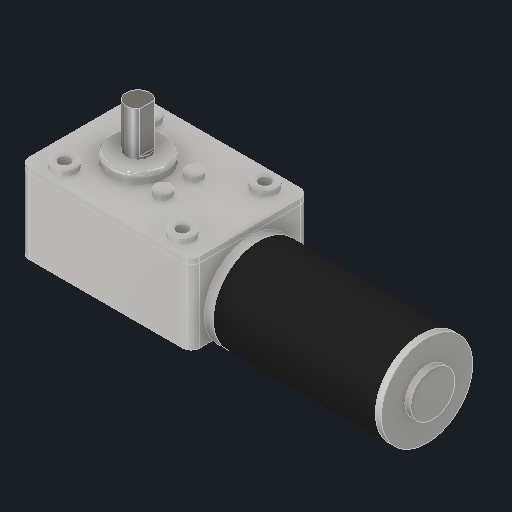
# Autodesk Inventor part: Worm_Gear_Motor_12V
Saved by Autodesk Inventor 2026.2 (Build 302298010, 298A)
## iProperties
Created: 2017-09-17
Part Number: Worm_Gear_Motor_12V
Material: Generic
Document SubType Name: Modeling
Designer: joeyt
Density: 1 g/cm^3
Appearance: Default
Author: joeyt
Autodesk Inventor part; units mm, degrees
ref_plane "YZ Plane" through (0, 0, 0) normal (1, 0, 0) x (0, 1, 0)
ref_plane "XZ Plane" through (0, 0, 0) normal (0, 1, 0) x (-1, 0, 0)
ref_plane "XY Plane" through (0, 0, 0) normal (0, 0, 1) x (1, 0, 0)
sketch "Sketch1" plane through (0, 0, 0) normal (0, 1, 0) x (-1, 0, 0)
  line L0 (-29, 20) -> (29, 20)
  line L1 (29, 20) -> (29, -20)
  line L2 (29, -20) -> (-29, -20)
  line L3 (-29, -20) -> (-29, 20)
  line L4 (-29, 20) -> (29, -20) construction
  line L5 (29, 20) -> (-29, -20) construction
  point P0 (0, 0)
  dimension "d0" = 58
  dimension "d1" = 40
  constraints: 12 end point, 2 midpoint, 2 parallel, 1 horizontal, 1 perpendicular
  measures "d0" distance of L1.end L2.end
  measures "d1" distance of L0.end L1.end
extrude "Extrusion1" add sketch "Sketch1" along normal blind 27
sketch "Sketch2" plane through (0, 27, 0) normal (0, 1, 0) x (1, 0, 0)
  line L0 (-29, 20) -> (-29, -20) projected
  line L1 (0, 0) -> (-29, 0)
  point P0 (-20, 14)
  point P1 (20, 14)
  point P2 (20, -14)
  point P3 (-20, -14)
  dimension "d4" = 40
  dimension "d5" = 28
  dimension "d6" = 9
  constraints: 2 end point, 2 horizontal alignment, 2 vertical alignment, 1 midpoint, 1 symmetric about line
  measures "d4" distance of point (20, 14) point (-20, 14)
  measures "d5" distance of point (-20, -14) point (-20, 14)
  measures "d6" distance from line of L0 point (-20, 14)
sketch "Sketch3" plane through (0, 27, 0) normal (0, 1, 0) x (1, 0, 0)
  circle A0 centre (-20, 14) radius 4
  circle A1 centre (-20, 14) radius 2
  point P0 (0, 0)
  dimension "d7" = 8
  dimension "d8" = 4
  constraints: 2 centre point, 2 coincident
  measures "d7" diameter of A0
  measures "d8" diameter of A1
extrude "Extrusion2" add sketch "Sketch3" along normal blind 2
sketch "Sketch11" plane through (-20, 27, -14) normal (0, 1, 0) x (1, 0, 0)
  circle A0 centre (0, 0) radius 2 projected
  point P0 (20, -14)
extrude "Extrusion9" cut sketch "Sketch11" against normal blind 10
pattern_sketch "Sketch Driven Pattern1" of "Extrusion2", "Extrusion9" from (-20, 27, -14) copies at (20, 27, -14) at (20, 27, 14) at (-20, 27, 14)
sketch "Sketch4" plane through (0, 27, 0) normal (0, 1, 0) x (1, 0, 0)
  circle A0 centre (-20, 14) radius 2 projected
  circle A1 centre (-20, -14) radius 2 projected
  circle A2 centre (-20, 14) radius 4 projected
  line L0 (-20, 14) -> (-20, -14)
  line L1 (-20, 0) -> (-9, 0)
  circle A3 centre (-9, 0) radius 9.5
  point P0 (0, 0)
  dimension "d11" = 11
  dimension "d12" = 19
  constraints: 4 end point, 1 centre point, 1 coincident, 1 horizontal, 1 midpoint, 1 vertical
  measures "d11" distance of L1.start L1.end
  measures "d12" diameter of A3
extrude "Extrusion3" add sketch "Sketch4" along normal blind 3.5 contours A3
sketch "Sketch9" plane through (0, 27, 0) normal (0, 1, 0) x (1, 0, 0)
  circle A0 centre (4.7197, 5.3096) radius 2.6969
  circle A1 centre (4.7197, -5.3096) radius 2.6969
  line L0 (0, 0) -> (14.4961, 0)
  constraints: 2 centre point, 2 end point, 1 equal radius, 1 horizontal, 1 symmetric about line
extrude "Extrusion8" add sketch "Sketch9" along normal blind 2
ref_plane "Work Plane1" through (0, 13.5, 0) normal (0, 1, 0) x (1, 0, 0)
thread "Thread1" size "M4x0.7" class "6H" standard "ANSI Metric M Profile" full length
thread "Thread2" size "8-32 UNC" class "2B" standard "ANSI Unified Screw Threads" full length
thread "Thread3" size "8-32 UNC" class "2B" standard "ANSI Unified Screw Threads" full length
thread "Thread4" size "8-32 UNC" class "2B" standard "ANSI Unified Screw Threads" full length
mirror "Mirror1" about plane through (0, 13.5, 0) normal (0, 1, 0) of "Extrusion3", "Extrusion2", "Sketch Driven Pattern1", "Extrusion8"
sketch "Sketch5" plane through (-9, 30.5, 0) normal (0, 1, 0) x (1, 0, 0)
  circle A0 centre (0, 0) radius 9.5 projected
  circle A1 centre (0, 0) radius 4
  point P0 (9, 0)
  dimension "d15" = 8
  constraints: 1 centre point, 1 coincident
  measures "d15" diameter of A1
extrude "Extrusion4" add sketch "Sketch5" along normal blind 15 separate body contours A1
sketch "Sketch6" plane through (-9, 45.5, 0) normal (0, 1, 0) x (1, 0, 0)
  circle A0 centre (0, 0) radius 4 projected
  circle A1 centre (0, 0) radius 9.5 projected
  circle A2 centre (-11, 14) radius 4 projected
  line L0 (-20, -20) -> (38, -20) projected
  line L1 (38, -20) -> (38, 20) projected
  line L2 (38, 20) -> (-20, 20) projected
  line L3 (-20, 20) -> (-20, -20) projected
  circle A3 centre (29, 14) radius 4 projected
  circle A4 centre (29, -14) radius 4 projected
  circle A5 centre (-11, -14) radius 4 projected
  line L4 (3, 4) -> (4, 4)
  line L5 (4, 4) -> (4, -4)
  line L6 (4, -4) -> (3, -4)
  line L7 (3, -4) -> (3, 4)
  circle A6 centre (0, 0) radius 4 projected
  point P0 (9, 0)
  dimension "d18" = 1
  constraints: 8 end point, 3 tangent, 2 parallel, 1 horizontal, 1 perpendicular
  measures "d18" distance between parallel lines of L5 L7
extrude "Extrusion5" cut sketch "Sketch6" against normal blind 14 contours A0 L7 | L5 L6 L7 A0 | A0 L7 L4 L5 picked at (3.1815, -0.6179) bodies 2
ref_plane "Work Plane2" through (0, 25, 0) normal (0, 1, 0) x (1, 0, 0)
fillet "Fillet1" radius 3 4 edges at (-29, 13.5, 20) (29, 13.5, 20) (29, 13.5, -20) (-29, 13.5, -20)
split body "Split1" result two bodies by plane through (0, 25, 0) normal (0, 1, 0) bodies 1 first body at (-6.1677, 25.5, 4.2246)
sketch "Sketch7" plane through (29, 0, 17) normal (1, 0, 0) x (0, 0, -1)
  circle A0 centre (17, 9) radius 15.5
  line L0 (34, 0) -> (0, 0) projected
  line L1 (0, 27) -> (34, 27) projected
  point P0 (17, 0)
  point P1 (17, 0)
  dimension "d23" = 31
  dimension "d24" = 18
  constraints: 1 centre point, 1 midpoint, 1 vertical alignment
  measures "d23" diameter of A0
  measures "d24" distance from line of A0.centre L1
extrude "Extrusion6" add sketch "Sketch7" along normal blind 62 separate body
sketch "Sketch8" plane through (91, 9, 0) normal (1, 0, 0) x (0, 0, -1)
  circle A0 centre (0, 0) radius 15.5 projected
  circle A1 centre (0, 0) radius 7.5
  point P0 (0, -9)
  dimension "d27" = 15
  constraints: 1 centre point, 1 coincident
  measures "d27" diameter of A1
extrude "Extrusion7" cut sketch "Sketch8" against normal blind 2 bodies 5
ref_plane "Work Plane3" through (87, 9, 0) normal (1, 0, 0) x (0, 0, -1)
ref_plane "Work Plane4" through (32, 0, 17) normal (1, 0, 0) x (0, 0, -1)
split_face "Split2"
split_face "Split3"
fillet "Fillet2" radius 1 2 edges at (-18.5, 30.5, 0) (-18.5, -3.5, 0)
sketch "Sketch12" plane through (0, 27, 0) normal (0, 1, 0) x (1, 0, 0)
  circle A0 centre (-9, 0) radius 4 projected
  circle A1 centre (-9, 0) radius 4
  point P0 (0, 0)
  constraints: 1 centre point, 1 coincident
body "Solid2"
body "Solid5"
body "Solid3"
body "Solid4"
